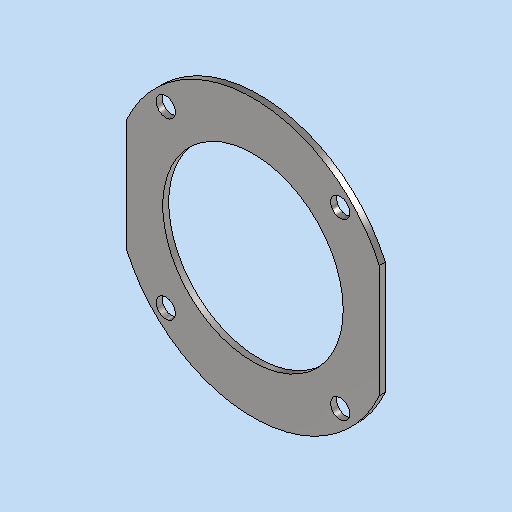
# Autodesk Inventor part: boron window
Saved by Autodesk Inventor 2025 (Build 290162000, 162)
## iProperties
Created: 2024-05-15
Part Number: boron window
Material: Stainless Steel
Document SubType Name: Modeling
Designer: queezz
Density: 8 g/cm^3
Appearance: Semi-Polished
Mass: 23.3231 g
Surface Area: 29.7529 cm^2
Volume: 2.91539 cm^3
Author: queezz
Autodesk Inventor part; units mm, degrees
ref_plane "YZ Plane" through (0, 0, 0) normal (1, 0, 0) x (0, 1, 0)
ref_plane "XZ Plane" through (0, 0, 0) normal (0, 1, 0) x (-1, 0, 0)
ref_plane "XY Plane" through (0, 0, 0) normal (0, 0, 1) x (1, 0, 0)
sketch "Sketch1" plane through (0, 0, 0) normal (0, 0, 1) x (1, 0, 0)
  circle A0 centre (0, 0) radius 15
  circle A1 centre (0, 0) radius 23
  dimension "d0" = 30
  dimension "d1" = 46
  constraints: 2 centre point, 2 coincident
  measures "d0" diameter of A0
  measures "d1" diameter of A1
extrude "Extrusion1" add sketch "Sketch1" along normal blind 1
sketch "Sketch2" plane through (0, 0, 1) normal (0, 0, 1) x (1, 0, 0)
  line L0 (0, 0) -> (23, 0) construction
  circle A0 centre (0, 0) radius 23 projected
  circle A1 centre (0, 0) radius 20.5 construction
  line L1 (0, 0) -> (14.4957, 14.4957) construction
  dimension "d35" = 41
  dimension "d34" = 45
  constraints: 4 end point, 2 coincident, 1 horizontal, 1 horizontal alignment, 4 other
  measures "d34" angle of L0 L1
hole "For-m3-screws" at (14.4957, 14.4957, 1) direction (0, 0, -1) diameter 3.2 end through all
pattern_circular "Circular Pattern1" count 4 over 360 about axis through (0, 0, 0) along (0, 0, 1) of "For-m3-screws"
sketch "Sketch4" plane through (0, 0, 0) normal (0, 0, 1) x (1, 0, 0)
  line L0 (21, 30) -> (26, 30)
  line L1 (26, 30) -> (26, -30)
  line L2 (26, -30) -> (21, -30)
  line L3 (21, -30) -> (21, 30)
  point P0 (0, 0)
  point P1 (26, 0)
  dimension "d19" = 21
  dimension "d20" = 60
  dimension "d21" = 5
  constraints: 8 end point, 2 parallel, 1 horizontal, 1 horizontal alignment, 1 midpoint, 1 perpendicular
  measures "d19" distance from line of L3 point (0, 0)
  measures "d20" distance of L0.end L1.end
  measures "d21" distance of L0.start L0.end
extrude "Extrusion3" cut sketch "Sketch4" along normal blind 10
mirror "Mirror1" about plane through (0, 0, 0) normal (1, 0, 0) of "Extrusion3"
equation "\"d0\" = innerdiameter"
equation "\"d1\" = outerdiameter"
equation "\"d35\" = holepositiondiameter"
equation "\"d19\" = trimspan"
equation "\"outerdiameter\" = 46"
equation "\"innerdiameter\" = 30"
equation "\"holepositiondiameter\" = 41"
equation "\"trimspan\" = 21"
body "Solid1"
